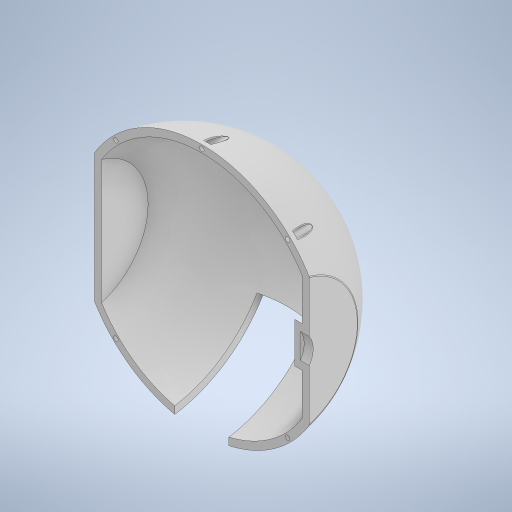
# Autodesk Inventor part: Head_front
Saved by Autodesk Inventor 2023.1 (Build 271208000, 208)
## iProperties
Created: 2022-08-09
Part Number: Head_front
Material: 일반
Document SubType Name: Modeling
Designer: fly01
Density: 1 g/cm^3
Appearance: 기본값
Author: fly01
Autodesk Inventor part; units mm, degrees
ref_plane "YZ Plane" through (0, 0, 0) normal (1, 0, 0) x (0, 1, 0)
ref_plane "XZ Plane" through (0, 0, 0) normal (0, 1, 0) x (-1, 0, 0)
sketch "스케치1" plane through (0, 0, 0) normal (0, 0, 1) x (1, 0, 0)
  line L0 (-42.5, 28) -> (42.5, 28)
  line L1 (42.5, 28) -> (42.5, -28)
  line L2 (42.5, -28) -> (-42.5, -28)
  line L3 (-42.5, -28) -> (-42.5, 28)
  line L4 (-42.5, 28) -> (42.5, -28) construction
  line L5 (42.5, 28) -> (-42.5, -28) construction
  circle A0 centre (0, 0) radius 70
  line L6 (42.5, -15.963) -> (59.5, -15.963)
  circle A1 centre (0, 0) radius 66
  line L7 (-70, 0) -> (70, 0)
  line L8 (0, 0) -> (0, 18.0759)
  line L9 (59.5, -36.8748) -> (59.5, 36.8748)
  line L10 (-59.5, -36.8748) -> (-59.5, 36.8748)
  point P0 (59.5, -28.5613)
  point P1 (59.5, 28.5613)
  point P2 (-59.5, -28.5613)
  point P3 (-59.5, 28.5613)
  point P4 (-59.5, 28.5613)
  point P5 (59.5, 0)
  point P6 (-59.5, 0)
  dimension "d0" = 85
  dimension "d1" = 56
  dimension "d2" = 17
  dimension "d3" = 140
  dimension "d4" = 4
  constraints: 22 end point, 8 point on circle, 5 point on line, 3 horizontal, 2 centre point, 2 midpoint, 2 parallel, 2 perpendicular, 2 symmetric about line, 1 coincident, 1 vertical
  measures "d0" distance of L0.start L0.end
  measures "d1" distance of L0.end L1.end
  measures "d2" distance of L6.start L6.end
  measures "d3" diameter of A0
  measures "d4" radial gap between concentric circles of A0 A1
revolve "회전1" add sketch "스케치1" angle 360 about axis through (-70, 0, 0) along (1, 0, 0) picked at (-51.0142, 43.6948) contours L3 L7 L10 A1 L9 L1 L0 | L0 L1 L7 L3 | L10 A0 L9 A1
ref_plane "작업 평면2" through (0, 0, -10) normal (0, 0, 1) x (1, 0, 0)
sketch "스케치16" plane through (0, 0, -10) normal (0, 0, 1) x (1, 0, 0)
  line L0 (-103.9396, 92.2366) -> (89.3759, 92.2366)
  line L1 (89.3759, 92.2366) -> (89.3759, -86.3418)
  line L2 (89.3759, -86.3418) -> (-103.9396, -86.3418)
  line L3 (-103.9396, -86.3418) -> (-103.9396, 92.2366)
  point P0 (0, 0)
  constraints: 8 end point, 2 parallel, 1 horizontal, 1 perpendicular
extrude "돌출14" cut sketch "스케치16" along normal blind 108
shell "쉘2" thickness 4 removed faces 1 at (-12.1927, -19.613, -10)
sketch "스케치17" plane through (0, 0, -10) normal (0, 0, 1) x (1, 0, 0)
  line L0 (-55.5, -34.2892) -> (-55.5, 34.2892) projected
  arc A0 (55.5, 34.2892) -> (-55.5, 34.2892) centre (0, 0) ccw projected
  line L1 (55.5, 34.2892) -> (55.5, -34.2892) projected
  arc A1 (-55.5, -34.2892) -> (55.5, -34.2892) centre (0, 0) ccw projected
  line L2 (-59.5, -35.493) -> (-59.5, 35.493) projected
  arc A2 (-59.5, -35.493) -> (59.5, -35.493) centre (0, 0) ccw projected
  line L3 (59.5, 35.493) -> (59.5, -35.493) projected
  arc A3 (59.5, 35.493) -> (-59.5, 35.493) centre (0, 0) ccw projected
  arc A4 (59.5, 35.493) -> (-59.5, 35.493) centre (0, 0) ccw projected
  line L4 (0, 69.282) -> (0, 65.238)
  circle A5 centre (0, 67.26) radius 1.25
  circle A6 centre (-47.56, 47.56) radius 1.25
  circle A7 centre (-67.26, 0) radius 1.25
  circle A8 centre (-47.56, -47.56) radius 1.25
  circle A9 centre (0, -67.26) radius 1.25
  circle A10 centre (47.56, -47.56) radius 1.25
  circle A11 centre (67.26, 0) radius 1.25
  circle A12 centre (47.56, 47.56) radius 1.25
  dimension "d72" = 2.5
  dimension "d75" = 360
  constraints: 8 centre point, 3 point on circle, 2 end point, 1 midpoint, 17 other
  measures "d72" diameter of A5
extrude "돌출15" cut sketch "스케치17" against normal blind 108 contours A5 L4 | L4 A5 | A6 | A8 | A9 | A10 | A12
ref_plane "작업 평면3" through (0, 0, -13) normal (0, 0, 1) x (1, 0, 0)
sketch "스케치18" plane through (0, 0, -13) normal (0, 0, 1) x (1, 0, 0)
  circle A0 centre (0, 67.26) radius 1.25 projected
  circle A1 centre (0, 67.26) radius 1.75
  circle A2 centre (-47.56, 47.56) radius 1.75
  circle A3 centre (-67.26, 0) radius 1.75
  circle A4 centre (-47.56, -47.56) radius 1.75
  circle A5 centre (0, -67.26) radius 1.75
  circle A6 centre (47.56, -47.56) radius 1.75
  circle A7 centre (67.26, 0) radius 1.75
  circle A8 centre (47.56, 47.56) radius 1.75
  point P0 (0, 0)
  point P1 (0, 0)
  point P2 (0, 0)
  point P3 (0, 0)
  point P4 (0, 0)
  point P5 (0, 0)
  point P6 (0, 0)
  point P7 (0, 0)
  dimension "d80" = 3.5
  dimension "d83" = 360
  constraints: 8 centre point, 3 coincident, 1 horizontal alignment, 24 other
  measures "d80" diameter of A1
extrude "돌출16" cut sketch "스케치18" against normal blind 108 contours A0 | A1 | A2 | A4 | A5 | A6 | A8
fillet "모깎기2" radius 0.5 12 edges at (1.5381, 68.0948, -16.1473) (-1.5496, 66.447, -21.9636) (49.2966, 47.7767, -13.6833) (45.9384, 46.902, -24.287) (-46.5764, 49.0074, -18.136) (-48.6486, 46.1898, -19.9954) (45.938, -46.9032, -24.2857) (49.2966, -47.7767, -13.6833) (-1.5499, -66.4475, -21.962) (1.5381, -68.0948, -16.1474) (-48.6488, -46.19, -19.9945) (-46.5764, -49.0074, -18.1359)
fillet "모깎기3" radius 1 2 edges at (59.5, 0, -36.8748) (-59.5, 0, -36.8748)
sketch "스케치19" plane through (0, 0, -10) normal (0, 0, 1) x (1, 0, 0)
  line L0 (-15, -32.26) -> (15, -32.26)
  line L1 (15, -32.26) -> (15, -102.26)
  line L2 (15, -102.26) -> (-15, -102.26)
  line L3 (-15, -102.26) -> (-15, -32.26)
  circle A0 centre (0, -67.26) radius 1.25 projected
  line L4 (-15, -32.26) -> (15, -102.26) construction
  line L5 (15, -32.26) -> (-15, -102.26) construction
  point P0 (0, 0)
  dimension "d89" = 30
  dimension "d90" = 70
  constraints: 12 end point, 2 midpoint, 2 parallel, 1 horizontal, 1 perpendicular
  measures "d89" distance of L1.end L2.end
  measures "d90" distance of L0.end L1.end
extrude "돌출17" cut sketch "스케치19" against normal blind 108
sketch "스케치20" plane through (59.5, 0, 0) normal (1, 0, 0) x (0, 0, -1)
  circle A0 centre (0, 0) radius 12.15
  dimension "d93" = 24.3
  constraints: 1 centre point, 1 coincident
  measures "d93" diameter of A0
sketch "스케치21" plane through (55.5, 0, 0) normal (-1, 0, 0) x (0, 0, 1)
  circle A0 centre (0, 0) radius 12.15
  circle A1 centre (0, 0) radius 15
  line L0 (-10, 35.1959) -> (-10, -35.1959) projected
  point P0 (-10, -6.9009)
  point P1 (-10, 6.9009)
  point P2 (-10, 11.1803)
  point P3 (-10, -11.1803)
  dimension "d94" = 24.3
  dimension "d95" = 30
  constraints: 2 centre point, 2 coincident
  measures "d94" diameter of A0
  measures "d95" diameter of A1
extrude "돌출18" add sketch "스케치21" along normal blind 1 contours A0 L0 A1 picked at (-13.9484, 0.4881)
extrude "돌출19" cut sketch "스케치20" against normal blind 4
sketch "스케치22" plane through (54.5, 0, 0) normal (-1, 0, 0) x (0, 0, 1)
  arc A0 (-10, 11.1803) -> (-10, -11.1803) centre (0, 0) ccw projected
  line L0 (-10, -6.9009) -> (-10, -35.1959) projected
  line L1 (-10, 14.3943) -> (-10, -6.9009)
  arc A1 (-10, 6.9009) -> (-10, -6.9009) centre (0, 0) ccw projected
  line L2 (-10, 6.9009) -> (-10, 11.1803) projected
  line L3 (-10, -11.1803) -> (-10, -6.9009) projected
  point P0 (-10, -8)
  point P1 (-10, 6.9009)
  constraints: 2 end point, 1 vertical
extrude "돌출20" add sketch "스케치22" along normal blind 3
